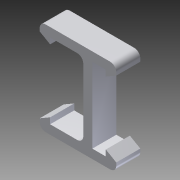
# Autodesk Inventor part: claw
Saved by Autodesk Inventor 2012 (Build 160160000, 160)
## iProperties
Created: 2014-07-18
Part Number: claw
Material: Default
Document SubType Name: Modeling
Designer: Anon
Density: 1 g/cm^3
Author: Anon
Autodesk Inventor part; units mm, degrees
ref_plane "YZ Plane" through (0, 0, 0) normal (1, 0, 0) x (0, 1, 0)
sketch "Sketch1" plane through (0, 0, 0) normal (0, 0, 1) x (1, 0, 0)
  line L0 (-12.5, -12) -> (12.5, -12)
  line L1 (12.5, -12) -> (12.5, -20)
  line L2 (12.5, -20) -> (-12.5, -20)
  line L3 (-12.5, -20) -> (-12.5, -12)
  point P0 (0, 0)
  dimension "d0" = 25
  dimension "d1" = 8
  dimension "d2" = 12.5
  dimension "d3" = 20
  constraints: 8 end point, 2 parallel, 1 horizontal, 1 perpendicular
  measures "d0" distance of L1.end L2.end
  measures "d1" distance of L0.end L1.end
  measures "d2" distance from line of point (0, 0) L3
  measures "d3" distance from line of point (0, 0) L2
extrude "Extrusion1" add sketch "Sketch1" along normal blind 3
sketch "Sketch3" plane through (-12.5, -20, 0) normal (0, -1, 0) x (1, 0, 0)
  line L0 (25, 3) -> (0, 3) projected
  line L1 (25, 0) -> (25, 3) projected
  line L2 (21.5359, 3) -> (21.5359, 5)
  line L3 (25, 3) -> (21.5359, 3)
  line L4 (25, 0) -> (0, 0) projected
  line L5 (21.5359, 5) -> (25, 3)
  point P0 (12.5, 0)
  dimension "d9" = 2
  dimension "d11" = 0
  dimension "d15" = 30
  constraints: 6 end point, 1 collinear, 1 parallel, 1 point on line
  measures "d9" distance of L2.start L2.end
  measures "d11" horizontal distance of L1.start L3.start
  measures "d15" angle of L4 L5
extrude "Extrusion2" add sketch "Sketch3" against normal blind 8
ref_plane "Work Plane1" through (4.5359, -20, 3) normal (-1, 0, 0) x (0, 0, 1)
sketch "Sketch4" plane through (4.5359, -20, 3) normal (-1, 0, 0) x (0, 0, 1)
  line L0 (0, 8) -> (12.5, 8)
  line L1 (12.5, 8) -> (12.5, 0)
  line L2 (12.5, 0) -> (0, 0)
  line L3 (0, 0) -> (0, 8)
  point P0 (-3, 20)
  dimension "d16" = 12.5
  dimension "d17" = 8
  dimension "d18" = 12
  dimension "d19" = 3
  constraints: 8 end point, 2 parallel, 1 horizontal, 1 perpendicular
  measures "d16" distance of L1.end L2.end
  measures "d17" distance of L0.end L1.end
  measures "d18" distance from line of L0 point (-3, 20)
  measures "d19" distance from line of L3 point (-3, 20)
extrude "Extrusion3" add sketch "Sketch4" along normal blind 3
ref_plane "Work Plane2" through (-9.4641, -20, 3) normal (-1, 0, 0) x (0, 0, 1)
sketch "Sketch5" plane through (-12.5, -20, 0) normal (0, -1, 0) x (1, 0, 0)
  line L0 (21.5359, 3) -> (17.0359, 3) projected
  line L1 (17.0359, 15.5) -> (17.0359, 3) projected
  line L2 (17.0359, 15.5) -> (14.0359, 15.5) projected
  line L3 (14.0359, 15.5) -> (14.0359, 3) projected
  line L4 (14.0359, 3) -> (0, 3) projected
  line L5 (0, 0) -> (0, 3) projected
  line L6 (25, 0) -> (0, 0) projected
  line L7 (25, 0) -> (25, 3) projected
  line L8 (21.5359, 5) -> (25, 3) projected
  line L9 (21.5359, 3) -> (21.5359, 5) projected
  line L10 (3.018, 3) -> (3.018, 5)
  line L11 (3.018, 5) -> (-0.4461, 3)
  line L12 (-0.4461, 3) -> (3.018, 3)
  line L13 (-0.4461, 3) -> (0, 3)
  line L14 (0, 3) -> (0, 0)
  line L15 (0, 0) -> (-0.4461, 0)
  line L16 (-0.4461, 0) -> (-0.4461, 3)
  point P0 (12.5, 0)
  dimension "d23" = 2
  dimension "d24" = 60
  constraints: 14 end point, 3 parallel, 2 point on line, 1 collinear, 1 horizontal, 1 perpendicular
  measures "d23" distance of L10.start L10.end
  measures "d24" angle of L11 L10
extrude "Extrusion4" add sketch "Sketch5" against normal blind 8
mirror "Mirror1" about plane through (4.5359, -12, 15.5) normal (0, 0, 1) of "Extrusion1", "Extrusion2", "Extrusion3", "Extrusion4"
fillet "Fillet1" radius 2 2 edges at (1.5359, -16, 28) (1.5359, -16, 3)
fillet "Fillet2" radius 2 4 edges at (-12.9461, -16, 31) (-12.9461, -16, 0) (12.5, -16, 31) (12.5, -16, 0)
ref_plane "Work Plane3" through (4.5359, -20, 28) normal (1, 0, 0) x (0, 0, -1)
ref_plane "Work Plane4" through (-9.4641, -20, 28) normal (1, 0, 0) x (0, 0, -1)
body "Solid1"
